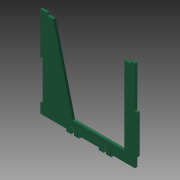
# Autodesk Inventor part: sideLeg
Saved by Autodesk Inventor 2015 SP1 (Build 190203100, 203)
## iProperties
Created: 2015-04-09
Part Number: sideLeg
Material: Generic
Document SubType Name: Modeling
Designer: Iain
Density: 1 g/cm^3
Appearance: Smooth - Dark Sea Green
Author: Iain
Autodesk Inventor part; units mm, degrees
sketch "Sketch1" plane through (0, 0, 0) normal (0, 1, 0) x (-1, 0, 0)
  line L0 (375, -351) -> (-375, -351)
  line L1 (-375, -351) -> (-375, 351)
  line L2 (-375, 351) -> (375, 351)
  line L3 (375, 351) -> (375, -351)
  point P0 (0, 0)
  point P1 (0, -351)
  point P2 (375, 0)
  dimension "d0" = 750
  dimension "d1" = 702
  constraints: 8 end point, 2 midpoint, 2 parallel, 1 horizontal, 1 horizontal alignment, 1 perpendicular, 1 vertical alignment
  measures "d0" distance of L0.start L0.end
  measures "d1" distance of L2.end L0.start
extrude "Extrusion1" add sketch "Sketch1" along normal blind 18
sketch "Sketch2" plane through (0, 18, 0) normal (0, 1, 0) x (1, 0, 0)
  line L0 (375, -351) -> (375, 351) construction
  line L1 (-375, 351) -> (375, 351) construction
  line L2 (375, 351) -> (375, 271) construction
  line L3 (375, 271) -> (-375, 271) construction
  line L4 (-375, 271) -> (-375, 351) construction
  line L5 (-375, -351) -> (-275, -351) construction
  line L6 (375, -351) -> (275, -351) construction
  line L7 (-375, -351) -> (375, -351) construction
  line L8 (-375, 271) -> (-125, 271) construction
  line L9 (-375, 351) -> (-375, -351) construction
  line L10 (-275, -351) -> (275, -351)
  line L11 (275, -351) -> (275, 271)
  line L12 (275, 271) -> (-125, 271)
  line L13 (-275, -351) -> (-275, -333)
  line L14 (-275, -333) -> (-125, 271)
  point P0 (0, 0)
  point P1 (375, 0)
  point P2 (-375, 0)
  point P3 (-250, 271)
  point P4 (0, 271)
  dimension "d4" = 80
  dimension "d5" = 100
  dimension "d6" = 100
  dimension "d7" = 250
  dimension "d101" = 18
  constraints: 24 end point, 4 horizontal, 4 midpoint, 2 collinear, 2 parallel, 2 perpendicular, 2 point on line, 2 vertical alignment, 1 coincident, 1 horizontal alignment, 1 vertical
  measures "d4" distance of L3.end L1.start
  measures "d5" distance of L5.start L5.end
  measures "d6" distance of L6.start L6.end
  measures "d7" distance of L8.start L8.end
  measures "d101" distance of L5.end L13.end
extrude "Extrusion2" cut sketch "Sketch2" against normal blind 18
sketch "Sketch3" plane through (0, 18, 0) normal (0, 1, 0) x (1, 0, 0)
  line L0 (-125, 271) -> (275, 271) projected
  line L1 (275, 271) -> (275, -351) projected
  line L2 (275, -351) -> (375, -351) projected
  line L3 (375, -351) -> (375, 351) projected
  line L4 (375, 351) -> (-375, 351) projected
  line L5 (-375, 351) -> (-375, -351) projected
  line L6 (-325, -333) -> (325, -333)
  line L7 (325, -333) -> (325, -351)
  line L8 (325, -351) -> (-325, -351)
  line L9 (-325, -351) -> (-325, -333)
  line L10 (275, -351) -> (375, -351) projected
  line L11 (-375, -351) -> (-275, -351) projected
  line L12 (-275, -351) -> (-275, -333) projected
  line L13 (-275, -333) -> (-125, 271) projected
  point P0 (0, 0)
  point P1 (0, -351)
  point P2 (325, -351)
  point P3 (325, -342)
  point P4 (325, -351)
  point P5 (-325, -342)
  point P6 (-325, -351)
  dimension "d11" = 18
  constraints: 8 end point, 5 midpoint, 2 parallel, 2 vertical alignment, 1 horizontal, 1 horizontal alignment, 1 perpendicular
  measures "d11" distance of L6.end L7.end
extrude "Extrusion3" cut sketch "Sketch3" against normal through all contours L12 L8 L9 L6 | L6 L1 L8 L12 | L6 L7 L2 L1
sketch "Sketch4" plane through (0, 18, 0) normal (0, 1, 0) x (1, 0, 0)
  line L0 (325, -333) -> (325, -351) projected
  line L1 (325, -351) -> (375, -351) projected
  line L2 (375, -351) -> (375, 351) projected
  line L3 (375, 351) -> (-375, 351) projected
  line L4 (-375, 351) -> (-375, -351) projected
  line L5 (-375, -351) -> (-325, -351) projected
  line L6 (-325, -351) -> (-325, -333) projected
  line L7 (-325, -333) -> (-275, -333) projected
  line L8 (-125, 271) -> (275, 271) projected
  line L9 (275, 271) -> (275, -333) projected
  line L10 (275, -333) -> (325, -333) projected
  line L11 (375, -31) -> (357, -31)
  line L12 (357, -31) -> (357, -351)
  line L13 (357, -351) -> (375, -351)
  line L14 (375, -351) -> (375, -31)
  line L15 (-275, -333) -> (-125, 271) projected
  point P0 (0, 0)
  point P1 (375, -191)
  point P2 (375, 0)
  point P3 (366, -351)
  point P4 (350, -351)
  point P5 (366, -31)
  point P6 (275, -31)
  dimension "d14" = 18
  constraints: 8 end point, 6 midpoint, 2 horizontal alignment, 2 parallel, 1 horizontal, 1 perpendicular, 1 vertical alignment
  measures "d14" distance of L11.start L11.end
extrude "Extrusion4" cut sketch "Sketch4" against normal through all contours L12 L11 L2 L1
sketch "Sketch5" plane through (0, 18, 0) normal (0, 1, 0) x (1, 0, 0)
  line L0 (375, 351) -> (357, 351)
  line L1 (357, 351) -> (357, 271)
  line L2 (357, 271) -> (375, 271)
  line L3 (375, 271) -> (375, 351)
  line L4 (357, -31) -> (375, -31) projected
  line L5 (375, -31) -> (375, 351) projected
  line L6 (375, 351) -> (-375, 351) projected
  line L7 (-375, 351) -> (-375, -351) projected
  line L8 (-375, -351) -> (-325, -351) projected
  line L9 (-325, -351) -> (-325, -333) projected
  line L10 (-325, -333) -> (-275, -333) projected
  line L11 (-125, 271) -> (275, 271) projected
  line L12 (275, 271) -> (275, -333) projected
  line L13 (275, -333) -> (325, -333) projected
  line L14 (325, -333) -> (325, -351) projected
  line L15 (325, -351) -> (357, -351) projected
  line L16 (357, -351) -> (357, -31) projected
  line L17 (-275, -333) -> (-125, 271) projected
  point P0 (0, 0)
  point P1 (375, 311)
  point P2 (375, 160)
  point P3 (366, 351)
  point P4 (0, 351)
  point P5 (366, 271)
  point P6 (75, 271)
  dimension "d17" = 18
  constraints: 8 end point, 6 midpoint, 2 horizontal alignment, 2 parallel, 1 horizontal, 1 perpendicular, 1 vertical alignment
  measures "d17" distance of L0.start L0.end
extrude "Extrusion5" cut sketch "Sketch5" against normal through all contours L3 L2 L1 L0
sketch "Sketch6" plane through (0, 18, 0) normal (0, 1, 0) x (1, 0, 0)
  line L0 (357, 271) -> (357, 351) projected
  line L1 (357, 351) -> (-375, 351) projected
  line L2 (-375, 351) -> (-375, -351) projected
  line L3 (-375, -351) -> (-325, -351) projected
  line L4 (-325, -351) -> (-325, -333) projected
  line L5 (-325, -333) -> (-275, -333) projected
  line L6 (-125, 271) -> (275, 271) projected
  line L7 (275, 271) -> (275, -333) projected
  line L8 (275, -333) -> (325, -333) projected
  line L9 (325, -333) -> (325, -351) projected
  line L10 (325, -351) -> (357, -351) projected
  line L11 (357, -351) -> (357, -31) projected
  line L12 (357, -31) -> (375, -31) projected
  line L13 (375, -31) -> (375, 271) projected
  line L14 (375, 271) -> (357, 271) projected
  line L15 (-375, 271) -> (-357, 271)
  line L16 (-357, 271) -> (-357, -31)
  line L17 (-357, -31) -> (-375, -31)
  line L18 (-375, -31) -> (-375, 271)
  line L19 (-275, -333) -> (-125, 271) projected
  point P0 (0, 0)
  point P1 (-375, 120)
  point P2 (-375, 0)
  point P3 (-366, 271)
  point P4 (75, 271)
  point P5 (-366, -31)
  point P6 (366, -31)
  dimension "d20" = 18
  constraints: 8 end point, 6 midpoint, 2 horizontal alignment, 2 parallel, 1 horizontal, 1 perpendicular, 1 vertical alignment
  measures "d20" distance of L15.start L15.end
extrude "Extrusion6" cut sketch "Sketch6" against normal through all contours L15 L16 L17 L2
fillet "Fillet1" radius 3.175 2 edges at (-125, 9, -271) (275, 9, -271)
sketch "Sketch7" plane through (0, 18, 0) normal (0, 1, 0) x (1, 0, 0)
  line L0 (-375, 271) -> (-357, 271) projected
  line L1 (-357, 271) -> (-357, -31) projected
  line L2 (-357, -31) -> (-375, -31) projected
  line L3 (-375, -31) -> (-375, -351) projected
  line L4 (-375, -351) -> (-325, -351) projected
  line L5 (-325, -351) -> (-325, -333) projected
  line L6 (-325, -333) -> (-275, -333) projected
  arc A0 (-122.517, 271) -> (-125.5984, 268.5902) centre (-122.517, 267.825) ccw projected
  line L7 (-122.517, 271) -> (271.825, 271) projected
  arc A1 (275, 267.825) -> (271.825, 271) centre (271.825, 267.825) ccw projected
  line L8 (275, 267.825) -> (275, -333) projected
  line L9 (275, -333) -> (325, -333) projected
  line L10 (325, -333) -> (325, -351) projected
  line L11 (325, -351) -> (357, -351) projected
  line L12 (357, -351) -> (357, -31) projected
  line L13 (357, -31) -> (375, -31) projected
  line L14 (375, -31) -> (375, 271) projected
  line L15 (375, 271) -> (357, 271) projected
  line L16 (357, 271) -> (357, 351) projected
  line L17 (357, 351) -> (-375, 351) projected
  line L18 (-375, 351) -> (-375, 271) projected
  line L19 (-175, 369) -> (-75, 369)
  line L20 (-75, 369) -> (-75, 351)
  line L21 (-75, 351) -> (-175, 351)
  line L22 (-175, 351) -> (-175, 369)
  line L23 (-275, -333) -> (-125.5984, 268.5902) projected
  point P0 (0, 0)
  point P1 (-125, 351)
  point P2 (-9, 351)
  dimension "d24" = 18
  dimension "d25" = 100
  dimension "d26" = 250
  constraints: 8 end point, 2 midpoint, 2 parallel, 1 horizontal, 1 horizontal alignment, 1 perpendicular
  measures "d24" distance of L19.end L20.end
  measures "d25" distance of L19.start L19.end
  measures "d26" distance of L17.end point (-125, 351)
extrude "Extrusion7" add sketch "Sketch7" against normal blind 18 contours L22 L19 L20 L17
ref_plane "Work Plane3" through (0, 0, -351) normal (-1, 0, 0) x (0, 0, 1)
mirror "Mirror3" about plane through (0, 0, -351) normal (-1, 0, 0) of "Extrusion7"
sketch "Sketch8" plane through (0, 18, 0) normal (0, 1, 0) x (1, 0, 0)
  line L0 (-134, 369) -> (-116, 369)
  line L1 (-116, 369) -> (-116, 320)
  line L2 (-116, 320) -> (-134, 320)
  line L3 (-134, 320) -> (-134, 369)
  line L4 (-375, 271) -> (-357, 271) projected
  line L5 (-357, 271) -> (-357, -31) projected
  line L6 (-357, -31) -> (-375, -31) projected
  line L7 (-375, -31) -> (-375, -351) projected
  line L8 (-375, -351) -> (-325, -351) projected
  line L9 (-325, -351) -> (-325, -333) projected
  line L10 (-325, -333) -> (-275, -333) projected
  arc A0 (-122.517, 271) -> (-125.5984, 268.5902) centre (-122.517, 267.825) ccw projected
  line L11 (-122.517, 271) -> (271.825, 271) projected
  arc A1 (275, 267.825) -> (271.825, 271) centre (271.825, 267.825) ccw projected
  line L12 (275, 267.825) -> (275, -333) projected
  line L13 (275, -333) -> (325, -333) projected
  line L14 (325, -333) -> (325, -351) projected
  line L15 (325, -351) -> (357, -351) projected
  line L16 (357, -351) -> (357, -31) projected
  line L17 (357, -31) -> (375, -31) projected
  line L18 (375, -31) -> (375, 271) projected
  line L19 (375, 271) -> (357, 271) projected
  line L20 (357, 271) -> (357, 351) projected
  line L21 (357, 351) -> (175, 351) projected
  line L22 (175, 351) -> (175, 369) projected
  line L23 (175, 369) -> (75, 369) projected
  line L24 (75, 369) -> (75, 351) projected
  line L25 (75, 351) -> (-75, 351) projected
  line L26 (-75, 369) -> (-75, 351) projected
  line L27 (-175, 369) -> (-75, 369) projected
  line L28 (-175, 351) -> (-175, 369) projected
  line L29 (-175, 351) -> (-375, 351) projected
  line L30 (-375, 351) -> (-375, 271) projected
  line L31 (-175, 369) -> (-75, 369) projected
  line L32 (271.825, 271) -> (-122.517, 271) construction
  line L33 (-275, -333) -> (-125.5984, 268.5902) projected
  point P0 (0, 0)
  point P1 (-125, 369)
  point P2 (-125, 369)
  point P3 (-125, 369)
  point P4 (-125, 320)
  point P5 (-75, 320)
  dimension "d29" = 18
  dimension "d32" = 49
  constraints: 8 end point, 4 midpoint, 2 coincident, 2 parallel, 1 horizontal, 1 horizontal alignment, 1 perpendicular
  measures "d29" distance of L0.start L0.end
  measures "d32" distance of L0.end L1.end
extrude "Extrusion8" cut sketch "Sketch8" against normal blind 18 contours L0 L1 L2 L3
mirror "Mirror4" about plane through (0, 0, -351) normal (-1, 0, 0) of "Extrusion8"
sketch "Sketch9" plane through (0, 18, 0) normal (0, 1, 0) x (1, 0, 0)
  line L0 (116, 320) -> (116, 369) projected
  line L1 (116, 369) -> (75, 369) projected
  line L2 (75, 369) -> (75, 351) projected
  line L3 (75, 351) -> (-75, 351) projected
  line L4 (-75, 369) -> (-75, 351) projected
  line L5 (-116, 369) -> (-75, 369) projected
  line L6 (-116, 369) -> (-116, 320) projected
  line L7 (-116, 320) -> (-134, 320) projected
  line L8 (-134, 320) -> (-134, 369) projected
  line L9 (-175, 369) -> (-134, 369) projected
  line L10 (-175, 351) -> (-175, 369) projected
  line L11 (-175, 351) -> (-375, 351) projected
  line L12 (-375, 351) -> (-375, 271) projected
  line L13 (-375, 271) -> (-357, 271) projected
  line L14 (-357, 271) -> (-357, -31) projected
  line L15 (-357, -31) -> (-375, -31) projected
  line L16 (-375, -31) -> (-375, -351) projected
  line L17 (-375, -351) -> (-325, -351) projected
  line L18 (-325, -351) -> (-325, -333) projected
  line L19 (-325, -333) -> (-275, -333) projected
  arc A0 (-122.517, 271) -> (-125.5984, 268.5902) centre (-122.517, 267.825) ccw projected
  line L20 (-122.517, 271) -> (271.825, 271) projected
  arc A1 (275, 267.825) -> (271.825, 271) centre (271.825, 267.825) ccw projected
  line L21 (275, 267.825) -> (275, -333) projected
  line L22 (275, -333) -> (325, -333) projected
  line L23 (325, -333) -> (325, -351) projected
  line L24 (325, -351) -> (357, -351) projected
  line L25 (357, -351) -> (357, -31) projected
  line L26 (357, -31) -> (375, -31) projected
  line L27 (375, -31) -> (375, 271) projected
  line L28 (375, 271) -> (357, 271) projected
  line L29 (357, 271) -> (357, 351) projected
  line L30 (357, 351) -> (175, 351) projected
  line L31 (175, 351) -> (175, 369) projected
  line L32 (175, 369) -> (134, 369) projected
  line L33 (134, 369) -> (134, 320) projected
  line L34 (134, 320) -> (116, 320) projected
  line L35 (-175, 351) -> (-178.175, 351) construction
  line L36 (-134, 323.175) -> (-134, 320) construction
  line L37 (-275, -333) -> (-125.5984, 268.5902) projected
  point P0 (0, 0)
  point P1 (-175, 360)
  point P2 (-176.5875, 351)
  point P3 (-275, 351)
  point P4 (-125, 320)
  point P5 (-134, 321.5875)
  point P6 (-134, 344.5)
  dimension "d33" = 3.175
  dimension "d34" = 3.175
  constraints: 6 midpoint, 4 end point, 2 coincident, 2 horizontal alignment, 2 vertical alignment, 1 horizontal, 1 vertical
  measures "d33" distance of L35.start L35.end
  measures "d34" distance of L36.start L36.end
hole "Hole1" at (-178.175, 18, -351) at (-134, 18, -323.175) direction (0, -1, 0) diameter 6.35 end through all
ref_plane "Work Plane4" through (-125, 18, -369) normal (-1, 0, 0) x (0, 0, 1)
mirror "Mirror5" about plane through (-125, 18, -369) normal (-1, 0, 0) of "Hole1"
mirror "Mirror6" about plane through (0, 0, -351) normal (-1, 0, 0) of "Hole1", "Mirror5"
sketch "Sketch10" plane through (0, 18, 0) normal (0, 1, 0) x (1, 0, 0)
  arc A0 (68.65, 351) -> (75, 351) centre (71.825, 351) ccw projected
  line L0 (68.65, 351) -> (-68.65, 351) projected
  arc A1 (-75, 351) -> (-68.65, 351) centre (-71.825, 351) ccw projected
  line L1 (-75, 369) -> (-75, 351) projected
  line L2 (-116, 369) -> (-75, 369) projected
  line L3 (-116, 369) -> (-116, 326.35) projected
  arc A2 (-116, 320) -> (-116, 326.35) centre (-116, 323.175) ccw projected
  line L4 (-116, 320) -> (-134, 320) projected
  arc A3 (-134, 326.35) -> (-134, 320) centre (-134, 323.175) ccw projected
  line L5 (-134, 326.35) -> (-134, 369) projected
  line L6 (-175, 369) -> (-134, 369) projected
  line L7 (-175, 351) -> (-175, 369) projected
  arc A4 (-181.35, 351) -> (-175, 351) centre (-178.175, 351) ccw projected
  line L8 (-181.35, 351) -> (-375, 351) projected
  line L9 (-375, 351) -> (-375, 271) projected
  line L10 (-375, 271) -> (-357, 271) projected
  line L11 (-357, 271) -> (-357, -31) projected
  line L12 (-357, -31) -> (-375, -31) projected
  line L13 (-375, -31) -> (-375, -351) projected
  line L14 (-375, -351) -> (-325, -351) projected
  line L15 (-325, -351) -> (-325, -333) projected
  line L16 (-325, -333) -> (-275, -333) projected
  arc A5 (-122.517, 271) -> (-125.5984, 268.5902) centre (-122.517, 267.825) ccw projected
  line L17 (-122.517, 271) -> (271.825, 271) projected
  arc A6 (275, 267.825) -> (271.825, 271) centre (271.825, 267.825) ccw projected
  line L18 (275, 267.825) -> (275, -333) projected
  line L19 (275, -333) -> (325, -333) projected
  line L20 (325, -333) -> (325, -351) projected
  line L21 (325, -351) -> (357, -351) projected
  line L22 (357, -351) -> (357, -31) projected
  line L23 (357, -31) -> (375, -31) projected
  line L24 (375, -31) -> (375, 271) projected
  line L25 (375, 271) -> (357, 271) projected
  line L26 (357, 271) -> (357, 351) projected
  line L27 (357, 351) -> (181.35, 351) projected
  arc A7 (175, 351) -> (181.35, 351) centre (178.175, 351) ccw projected
  line L28 (175, 351) -> (175, 369) projected
  line L29 (175, 369) -> (134, 369) projected
  line L30 (134, 369) -> (134, 326.35) projected
  arc A8 (134, 320) -> (134, 326.35) centre (134, 323.175) ccw projected
  line L31 (134, 320) -> (116, 320) projected
  arc A9 (116, 326.35) -> (116, 320) centre (116, 323.175) ccw projected
  line L32 (116, 326.35) -> (116, 369) projected
  line L33 (116, 369) -> (75, 369) projected
  line L34 (75, 369) -> (75, 351) projected
  line L35 (-275, -333) -> (-125.5984, 268.5902) projected
  point P0 (0, 0)
  point P1 (-357, 267.825)
  dimension "d42" = 3.175
  constraints: 1 vertical alignment
  measures "d42" distance from line of L10 point (-357, 267.825)
hole "Hole2" at (-357, 18, -267.825) direction (0, -1, 0) diameter 6.35 end through all
ref_plane "Work Plane5" through (-375, 0, -120) normal (0, 0, 1) x (1, 0, 0)
mirror "Mirror7" about plane through (-375, 0, -120) normal (0, 0, 1) of "Hole2"
sketch "Sketch11" plane through (0, 18, 0) normal (0, 1, 0) x (1, 0, 0)
  arc A0 (-357, -31) -> (-357, -24.65) centre (-357, -27.825) ccw projected
  line L0 (-357, -31) -> (-375, -31) projected
  line L1 (-375, -31) -> (-375, -351) projected
  line L2 (-375, -351) -> (-325, -351) projected
  line L3 (-325, -351) -> (-325, -333) projected
  line L4 (-325, -333) -> (-275, -333) projected
  arc A1 (-122.517, 271) -> (-125.5984, 268.5902) centre (-122.517, 267.825) ccw projected
  line L5 (-122.517, 271) -> (271.825, 271) projected
  arc A2 (275, 267.825) -> (271.825, 271) centre (271.825, 267.825) ccw projected
  line L6 (275, 267.825) -> (275, -333) projected
  line L7 (275, -333) -> (325, -333) projected
  line L8 (325, -333) -> (325, -351) projected
  line L9 (325, -351) -> (357, -351) projected
  line L10 (357, -351) -> (357, -31) projected
  line L11 (357, -31) -> (375, -31) projected
  line L12 (375, -31) -> (375, 271) projected
  line L13 (375, 271) -> (357, 271) projected
  line L14 (357, 271) -> (357, 351) projected
  line L15 (357, 351) -> (181.35, 351) projected
  arc A3 (175, 351) -> (181.35, 351) centre (178.175, 351) ccw projected
  line L16 (175, 351) -> (175, 369) projected
  line L17 (175, 369) -> (134, 369) projected
  line L18 (134, 369) -> (134, 326.35) projected
  arc A4 (134, 320) -> (134, 326.35) centre (134, 323.175) ccw projected
  line L19 (134, 320) -> (116, 320) projected
  arc A5 (116, 326.35) -> (116, 320) centre (116, 323.175) ccw projected
  line L20 (116, 326.35) -> (116, 369) projected
  line L21 (116, 369) -> (75, 369) projected
  line L22 (75, 369) -> (75, 351) projected
  arc A6 (68.65, 351) -> (75, 351) centre (71.825, 351) ccw projected
  line L23 (68.65, 351) -> (-68.65, 351) projected
  arc A7 (-75, 351) -> (-68.65, 351) centre (-71.825, 351) ccw projected
  line L24 (-75, 369) -> (-75, 351) projected
  line L25 (-116, 369) -> (-75, 369) projected
  line L26 (-116, 369) -> (-116, 326.35) projected
  arc A8 (-116, 320) -> (-116, 326.35) centre (-116, 323.175) ccw projected
  line L27 (-116, 320) -> (-134, 320) projected
  arc A9 (-134, 326.35) -> (-134, 320) centre (-134, 323.175) ccw projected
  line L28 (-134, 326.35) -> (-134, 369) projected
  line L29 (-175, 369) -> (-134, 369) projected
  line L30 (-175, 351) -> (-175, 369) projected
  arc A10 (-181.35, 351) -> (-175, 351) centre (-178.175, 351) ccw projected
  line L31 (-181.35, 351) -> (-375, 351) projected
  line L32 (-375, 351) -> (-375, 271) projected
  line L33 (-375, 271) -> (-357, 271) projected
  arc A11 (-357, 264.65) -> (-357, 271) centre (-357, 267.825) ccw projected
  line L34 (-357, 264.65) -> (-357, -24.65) projected
  line L35 (-275, -333) -> (-125.5984, 268.5902) projected
  point P0 (0, 0)
  point P1 (357, 274.175)
  dimension "d50" = 3.175
  constraints: 1 vertical alignment
  measures "d50" distance of L13.end point (357, 274.175)
hole "Hole3" at (357, 18, -274.175) direction (0, -1, 0) diameter 6.35 end through all
mirror "Mirror8" about plane through (-375, 0, -120) normal (0, 0, 1) of "Hole3"
sketch "Sketch12" plane through (0, 18, 0) normal (0, 1, 0) x (1, 0, 0)
  arc A0 (357, -31) -> (357, -37.35) centre (357, -34.175) ccw projected
  line L0 (357, -31) -> (375, -31) projected
  line L1 (375, -31) -> (375, 271) projected
  line L2 (375, 271) -> (357, 271) projected
  arc A1 (357, 277.35) -> (357, 271) centre (357, 274.175) ccw projected
  line L3 (357, 277.35) -> (357, 351) projected
  line L4 (357, 351) -> (181.35, 351) projected
  arc A2 (175, 351) -> (181.35, 351) centre (178.175, 351) ccw projected
  line L5 (175, 351) -> (175, 369) projected
  line L6 (175, 369) -> (134, 369) projected
  line L7 (134, 369) -> (134, 326.35) projected
  arc A3 (134, 320) -> (134, 326.35) centre (134, 323.175) ccw projected
  line L8 (134, 320) -> (116, 320) projected
  arc A4 (116, 326.35) -> (116, 320) centre (116, 323.175) ccw projected
  line L9 (116, 326.35) -> (116, 369) projected
  line L10 (116, 369) -> (75, 369) projected
  line L11 (75, 369) -> (75, 351) projected
  arc A5 (68.65, 351) -> (75, 351) centre (71.825, 351) ccw projected
  line L12 (68.65, 351) -> (-68.65, 351) projected
  arc A6 (-75, 351) -> (-68.65, 351) centre (-71.825, 351) ccw projected
  line L13 (-75, 369) -> (-75, 351) projected
  line L14 (-116, 369) -> (-75, 369) projected
  line L15 (-116, 369) -> (-116, 326.35) projected
  arc A7 (-116, 320) -> (-116, 326.35) centre (-116, 323.175) ccw projected
  line L16 (-116, 320) -> (-134, 320) projected
  arc A8 (-134, 326.35) -> (-134, 320) centre (-134, 323.175) ccw projected
  line L17 (-134, 326.35) -> (-134, 369) projected
  line L18 (-175, 369) -> (-134, 369) projected
  line L19 (-175, 351) -> (-175, 369) projected
  arc A9 (-181.35, 351) -> (-175, 351) centre (-178.175, 351) ccw projected
  line L20 (-181.35, 351) -> (-375, 351) projected
  line L21 (-375, 351) -> (-375, 271) projected
  line L22 (-375, 271) -> (-357, 271) projected
  arc A10 (-357, 264.65) -> (-357, 271) centre (-357, 267.825) ccw projected
  line L23 (-357, 264.65) -> (-357, -24.65) projected
  arc A11 (-357, -31) -> (-357, -24.65) centre (-357, -27.825) ccw projected
  line L24 (-357, -31) -> (-375, -31) projected
  line L25 (-375, -31) -> (-375, -351) projected
  line L26 (-375, -351) -> (-325, -351) projected
  line L27 (-325, -351) -> (-325, -333) projected
  line L28 (-325, -333) -> (-275, -333) projected
  arc A12 (-122.517, 271) -> (-125.5984, 268.5902) centre (-122.517, 267.825) ccw projected
  line L29 (-122.517, 271) -> (271.825, 271) projected
  arc A13 (275, 267.825) -> (271.825, 271) centre (271.825, 267.825) ccw projected
  line L30 (275, 267.825) -> (275, -333) projected
  line L31 (275, -333) -> (325, -333) projected
  line L32 (325, -333) -> (325, -351) projected
  line L33 (325, -351) -> (357, -351) projected
  line L34 (357, -351) -> (357, -37.35) projected
  line L35 (-275, -333) -> (-125.5984, 268.5902) projected
  point P0 (0, 0)
  point P1 (-321.825, -333)
  dimension "d58" = 3.175
  constraints: 1 horizontal alignment
  measures "d58" distance of point (-321.825, -333) L27.end
hole "Hole4" at (-321.825, 18, 333) direction (0, -1, 0) diameter 6.35 end through all
mirror "Mirror9" about plane through (0, 0, -351) normal (-1, 0, 0) of "Hole4"
sketch "Sketch13" plane through (0, 18, 0) normal (0, 1, 0) x (1, 0, 0)
  arc A0 (325, -333) -> (318.65, -333) centre (321.825, -333) ccw projected
  line L0 (325, -333) -> (325, -351) projected
  line L1 (325, -351) -> (357, -351) projected
  line L2 (357, -351) -> (357, -37.35) projected
  arc A1 (357, -31) -> (357, -37.35) centre (357, -34.175) ccw projected
  line L3 (357, -31) -> (375, -31) projected
  line L4 (375, -31) -> (375, 271) projected
  line L5 (375, 271) -> (357, 271) projected
  arc A2 (357, 277.35) -> (357, 271) centre (357, 274.175) ccw projected
  line L6 (357, 277.35) -> (357, 351) projected
  line L7 (357, 351) -> (181.35, 351) projected
  arc A3 (175, 351) -> (181.35, 351) centre (178.175, 351) ccw projected
  line L8 (175, 351) -> (175, 369) projected
  line L9 (175, 369) -> (134, 369) projected
  line L10 (134, 369) -> (134, 326.35) projected
  arc A4 (134, 320) -> (134, 326.35) centre (134, 323.175) ccw projected
  line L11 (134, 320) -> (116, 320) projected
  arc A5 (116, 326.35) -> (116, 320) centre (116, 323.175) ccw projected
  line L12 (116, 326.35) -> (116, 369) projected
  line L13 (116, 369) -> (75, 369) projected
  line L14 (75, 369) -> (75, 351) projected
  arc A6 (68.65, 351) -> (75, 351) centre (71.825, 351) ccw projected
  line L15 (68.65, 351) -> (-68.65, 351) projected
  arc A7 (-75, 351) -> (-68.65, 351) centre (-71.825, 351) ccw projected
  line L16 (-75, 369) -> (-75, 351) projected
  line L17 (-116, 369) -> (-75, 369) projected
  line L18 (-116, 369) -> (-116, 326.35) projected
  arc A8 (-116, 320) -> (-116, 326.35) centre (-116, 323.175) ccw projected
  line L19 (-116, 320) -> (-134, 320) projected
  arc A9 (-134, 326.35) -> (-134, 320) centre (-134, 323.175) ccw projected
  line L20 (-134, 326.35) -> (-134, 369) projected
  line L21 (-175, 369) -> (-134, 369) projected
  line L22 (-175, 351) -> (-175, 369) projected
  arc A10 (-181.35, 351) -> (-175, 351) centre (-178.175, 351) ccw projected
  line L23 (-181.35, 351) -> (-375, 351) projected
  line L24 (-375, 351) -> (-375, 271) projected
  line L25 (-375, 271) -> (-357, 271) projected
  arc A11 (-357, 264.65) -> (-357, 271) centre (-357, 267.825) ccw projected
  line L26 (-357, 264.65) -> (-357, -24.65) projected
  arc A12 (-357, -31) -> (-357, -24.65) centre (-357, -27.825) ccw projected
  line L27 (-357, -31) -> (-375, -31) projected
  line L28 (-375, -31) -> (-375, -351) projected
  line L29 (-375, -351) -> (-325, -351) projected
  line L30 (-325, -351) -> (-325, -333) projected
  arc A13 (-318.65, -333) -> (-325, -333) centre (-321.825, -333) ccw projected
  line L31 (-318.65, -333) -> (-275, -333) projected
  arc A14 (-122.517, 271) -> (-125.5984, 268.5902) centre (-122.517, 267.825) ccw projected
  line L32 (-122.517, 271) -> (271.825, 271) projected
  arc A15 (275, 267.825) -> (271.825, 271) centre (271.825, 267.825) ccw projected
  line L33 (275, 267.825) -> (275, -333) projected
  line L34 (275, -333) -> (318.65, -333) projected
  line L35 (-275, -333) -> (-125.5984, 268.5902) projected
  point P0 (0, 0)
  point P1 (-366, -182)
  dimension "d66" = 302
  dimension "d67" = 151
  dimension "d68" = 9
  measures "d66" vertical distance of L31.start L27.end
  measures "d67" vertical distance of point (-366, -182) L27.end
  measures "d68" distance from line of L28 point (-366, -182)
hole "Hole5" at (-366, 18, 182) direction (0, -1, 0) diameter 6.35 end through all
sketch "Sketch14" plane through (0, 18, 0) normal (0, 1, 0) x (1, 0, 0)
  circle A0 centre (-366, -182) radius 3.175 projected
  arc A1 (325, -333) -> (318.65, -333) centre (321.825, -333) ccw projected
  line L0 (325, -333) -> (325, -351) projected
  line L1 (325, -351) -> (357, -351) projected
  line L2 (357, -351) -> (357, -37.35) projected
  arc A2 (357, -31) -> (357, -37.35) centre (357, -34.175) ccw projected
  line L3 (357, -31) -> (375, -31) projected
  line L4 (375, -31) -> (375, 271) projected
  line L5 (375, 271) -> (357, 271) projected
  arc A3 (357, 277.35) -> (357, 271) centre (357, 274.175) ccw projected
  line L6 (357, 277.35) -> (357, 351) projected
  line L7 (357, 351) -> (181.35, 351) projected
  arc A4 (175, 351) -> (181.35, 351) centre (178.175, 351) ccw projected
  line L8 (175, 351) -> (175, 369) projected
  line L9 (175, 369) -> (134, 369) projected
  line L10 (134, 369) -> (134, 326.35) projected
  arc A5 (134, 320) -> (134, 326.35) centre (134, 323.175) ccw projected
  line L11 (134, 320) -> (116, 320) projected
  arc A6 (116, 326.35) -> (116, 320) centre (116, 323.175) ccw projected
  line L12 (116, 326.35) -> (116, 369) projected
  line L13 (116, 369) -> (75, 369) projected
  line L14 (75, 369) -> (75, 351) projected
  arc A7 (68.65, 351) -> (75, 351) centre (71.825, 351) ccw projected
  line L15 (68.65, 351) -> (-68.65, 351) projected
  arc A8 (-75, 351) -> (-68.65, 351) centre (-71.825, 351) ccw projected
  line L16 (-75, 369) -> (-75, 351) projected
  line L17 (-116, 369) -> (-75, 369) projected
  line L18 (-116, 369) -> (-116, 326.35) projected
  arc A9 (-116, 320) -> (-116, 326.35) centre (-116, 323.175) ccw projected
  line L19 (-116, 320) -> (-134, 320) projected
  arc A10 (-134, 326.35) -> (-134, 320) centre (-134, 323.175) ccw projected
  line L20 (-134, 326.35) -> (-134, 369) projected
  line L21 (-175, 369) -> (-134, 369) projected
  line L22 (-175, 351) -> (-175, 369) projected
  arc A11 (-181.35, 351) -> (-175, 351) centre (-178.175, 351) ccw projected
  line L23 (-181.35, 351) -> (-375, 351) projected
  line L24 (-375, 351) -> (-375, 271) projected
  line L25 (-375, 271) -> (-357, 271) projected
  arc A12 (-357, 264.65) -> (-357, 271) centre (-357, 267.825) ccw projected
  line L26 (-357, 264.65) -> (-357, -24.65) projected
  arc A13 (-357, -31) -> (-357, -24.65) centre (-357, -27.825) ccw projected
  line L27 (-357, -31) -> (-375, -31) projected
  line L28 (-375, -31) -> (-375, -351) projected
  line L29 (-375, -351) -> (-325, -351) projected
  line L30 (-325, -351) -> (-325, -333) projected
  arc A14 (-318.65, -333) -> (-325, -333) centre (-321.825, -333) ccw projected
  line L31 (-318.65, -333) -> (-275, -333) projected
  arc A15 (-122.517, 271) -> (-125.5984, 268.5902) centre (-122.517, 267.825) ccw projected
  line L32 (-122.517, 271) -> (271.825, 271) projected
  arc A16 (275, 267.825) -> (271.825, 271) centre (271.825, 267.825) ccw projected
  line L33 (275, 267.825) -> (275, -333) projected
  line L34 (275, -333) -> (318.65, -333) projected
  line L35 (-275, -333) -> (-125.5984, 268.5902) projected
  point P0 (0, 0)
  point P1 (-366, 311)
  point P2 (-375, 311)
  dimension "d76" = 9
  constraints: 1 horizontal alignment, 1 midpoint
  measures "d76" distance of point (-375, 311) point (-366, 311)
hole "Hole6" at (-366, 18, -311) direction (0, -1, 0) diameter 6.35 end through all
sketch "Sketch15" plane through (0, 18, 0) normal (0, 1, 0) x (1, 0, 0)
  line L0 (-125, 271) -> (-125, 320) construction
  line L1 (271.825, 271) -> (-122.517, 271) construction
  line L2 (-116, 320) -> (-134, 320) construction
  point P0 (0, 0)
  point P1 (-125, 295.5)
  point P2 (-125, 295.5)
  dimension "d84" = 49
  constraints: 3 midpoint, 2 coincident, 2 end point, 1 perpendicular, 1 vertical alignment
  measures "d84" distance of L0.start L0.end
hole "Hole7" at (-125, 18, -295.5) direction (0, -1, 0) diameter 6.35 end through all
mirror "Mirror10" about plane through (0, 0, -351) normal (-1, 0, 0) of "Hole7"
sketch "Sketch16" plane through (0, 18, 0) normal (0, 1, 0) x (1, 0, 0)
  circle A0 centre (125, 295.5) radius 3.175 projected
  circle A1 centre (-125, 295.5) radius 3.175 projected
  circle A2 centre (-366, 311) radius 3.175 projected
  circle A3 centre (-366, -182) radius 3.175 projected
  arc A4 (325, -333) -> (318.65, -333) centre (321.825, -333) ccw projected
  line L0 (325, -333) -> (325, -351) projected
  line L1 (325, -351) -> (357, -351) projected
  line L2 (357, -351) -> (357, -37.35) projected
  arc A5 (357, -31) -> (357, -37.35) centre (357, -34.175) ccw projected
  line L3 (357, -31) -> (375, -31) projected
  line L4 (375, -31) -> (375, 271) projected
  line L5 (375, 271) -> (357, 271) projected
  arc A6 (357, 277.35) -> (357, 271) centre (357, 274.175) ccw projected
  line L6 (357, 277.35) -> (357, 351) projected
  line L7 (357, 351) -> (181.35, 351) projected
  arc A7 (175, 351) -> (181.35, 351) centre (178.175, 351) ccw projected
  line L8 (175, 351) -> (175, 369) projected
  line L9 (175, 369) -> (134, 369) projected
  line L10 (134, 369) -> (134, 326.35) projected
  arc A8 (134, 320) -> (134, 326.35) centre (134, 323.175) ccw projected
  line L11 (134, 320) -> (116, 320) projected
  arc A9 (116, 326.35) -> (116, 320) centre (116, 323.175) ccw projected
  line L12 (116, 326.35) -> (116, 369) projected
  line L13 (116, 369) -> (75, 369) projected
  line L14 (75, 369) -> (75, 351) projected
  arc A10 (68.65, 351) -> (75, 351) centre (71.825, 351) ccw projected
  line L15 (68.65, 351) -> (-68.65, 351) projected
  arc A11 (-75, 351) -> (-68.65, 351) centre (-71.825, 351) ccw projected
  line L16 (-75, 369) -> (-75, 351) projected
  line L17 (-116, 369) -> (-75, 369) projected
  line L18 (-116, 369) -> (-116, 326.35) projected
  arc A12 (-116, 320) -> (-116, 326.35) centre (-116, 323.175) ccw projected
  line L19 (-116, 320) -> (-134, 320) projected
  arc A13 (-134, 326.35) -> (-134, 320) centre (-134, 323.175) ccw projected
  line L20 (-134, 326.35) -> (-134, 369) projected
  line L21 (-175, 369) -> (-134, 369) projected
  line L22 (-175, 351) -> (-175, 369) projected
  arc A14 (-181.35, 351) -> (-175, 351) centre (-178.175, 351) ccw projected
  line L23 (-181.35, 351) -> (-375, 351) projected
  line L24 (-375, 351) -> (-375, 271) projected
  line L25 (-375, 271) -> (-357, 271) projected
  arc A15 (-357, 264.65) -> (-357, 271) centre (-357, 267.825) ccw projected
  line L26 (-357, 264.65) -> (-357, -24.65) projected
  arc A16 (-357, -31) -> (-357, -24.65) centre (-357, -27.825) ccw projected
  line L27 (-357, -31) -> (-375, -31) projected
  line L28 (-375, -31) -> (-375, -351) projected
  line L29 (-375, -351) -> (-325, -351) projected
  line L30 (-325, -351) -> (-325, -333) projected
  arc A17 (-318.65, -333) -> (-325, -333) centre (-321.825, -333) ccw projected
  line L31 (-318.65, -333) -> (-275, -333) projected
  arc A18 (-122.517, 271) -> (-125.5984, 268.5902) centre (-122.517, 267.825) ccw projected
  line L32 (-122.517, 271) -> (271.825, 271) projected
  arc A19 (275, 267.825) -> (271.825, 271) centre (271.825, 267.825) ccw projected
  line L33 (275, 267.825) -> (275, -333) projected
  line L34 (275, -333) -> (318.65, -333) projected
  line L35 (-275, -333) -> (-125.5984, 268.5902) projected
  point P0 (0, 0)
  point P1 (366, 120)
  point P2 (375, 120)
  dimension "d92" = 9
  constraints: 1 horizontal alignment, 1 midpoint
  measures "d92" distance of point (375, 120) point (366, 120)
hole "Hole8" at (366, 18, -120) direction (0, -1, 0) diameter 6.35 end through all
fillet "Fillet2" radius 3.175 4 edges at (-375, 9, -271) (-375, 9, 31) (375, 9, -271) (375, 9, 31)
equation "\"d0\" = tableWidth"
equation "\"d1\" = legHeight"
equation "\"d2\" = plyThickness"
equation "\"d4\" = legTopDepth"
equation "\"d5\" = legBaseWidth"
equation "\"d6\" = legBaseWidth"
equation "\"d7\" = legTopWidthLong"
equation "\"d101\" = plyThickness"
equation "\"d8\" = temp"
equation "\"d11\" = plyThickness"
equation "\"d14\" = plyThickness"
equation "\"d17\" = plyThickness"
equation "\"d20\" = plyThickness"
equation "\"d23\" = 0.5 * millDiameter"
equation "\"d24\" = legTopTabHeight"
equation "\"d25\" = legTabTotalWidth"
equation "\"d26\" = 0.333333 * tableWidth"
equation "\"d27\" = plyThickness"
equation "\"d29\" = plyThickness"
equation "\"d32\" = legTopSlotDepth"
equation "\"d30\" = plyThickness"
equation "\"d33\" = 0.5 * millDiameter"
equation "\"d34\" = 0.5 * millDiameter"
equation "\"d35\" = millDiameter"
equation "\"d42\" = 0.5 * millDiameter"
equation "\"d43\" = millDiameter"
equation "\"d50\" = 0.5 * millDiameter"
equation "\"d51\" = millDiameter"
equation "\"d58\" = 0.5 * millDiameter"
equation "\"d59\" = millDiameter"
equation "\"d67\" = 0.5 * d66"
equation "\"d68\" = 0.5 * plyThickness"
equation "\"d69\" = millDiameter"
equation "\"d76\" = 0.5 * plyThickness"
equation "\"d77\" = millDiameter"
equation "\"d84\" = legTopSlotDepth"
equation "\"d85\" = millDiameter"
equation "\"d92\" = 0.5 * plyThickness"
equation "\"d93\" = millDiameter"
equation "\"d100\" = 0.5 * millDiameter"
equation "\"temp\" = 18"
equation "\"plyThickness\" = 18"
equation "\"legHeight\" = 702"
equation "\"tableWidth\" = 750"
equation "\"legBaseWidth\" = 100"
equation "\"legTopWidthLong\" = 250"
equation "\"legTopDepth\" = 80"
equation "\"millDiameter\" = 6.35"
equation "\"legTopTabHeight\" = 18"
equation "\"legTabTotalWidth\" = 100"
equation "\"legTopSlotDepth\" = 49"
body "Solid1"
